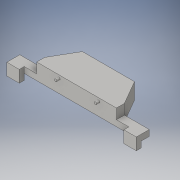
# Autodesk Inventor part: LED_Holder_V1
Saved by Autodesk Inventor 2016 (Build 200138000, 138)
## iProperties
Created: 2016-01-19
Part Number: LED_Holder_V1
Material: Generic
Document SubType Name: Modeling
Designer: Alexis Renderos
Density: 1 g/cm^3
Appearance: Default
Author: Alexis Renderos
Autodesk Inventor part; units mm, degrees
ref_plane "YZ Plane" through (0, 0, 0) normal (1, 0, 0) x (0, 1, 0)
ref_plane "XZ Plane" through (0, 0, 0) normal (0, 1, 0) x (-1, 0, 0)
ref_plane "XY Plane" through (0, 0, 0) normal (0, 0, 1) x (1, 0, 0)
sketch "Sketch1" plane through (0, 0, 0) normal (0, 0, 1) x (1, 0, 0)
  line L0 (0, 12.3444) -> (0, -2.0574) projected
  line L1 (-35.56, 0) -> (35.56, 0) projected
  line L2 (-35.56, 0) -> (35.56, 0) projected
  line L3 (0, -2.0574) -> (0, 12.3444) projected
  line L4 (-12.319, 8.2169) -> (15.113, 8.2169)
  line L5 (-10.2108, 8.2169) -> (13.0048, 8.2169)
  circle A0 centre (-11.2649, 8.2169) radius 1.0541
  circle A1 centre (14.0589, 8.2169) radius 1.0541
  line L6 (-25.4, 10.287) -> (-25.4, 0)
  line L7 (-25.4, 0) -> (25.4, 0)
  line L8 (-25.4, 10.287) -> (25.4, 10.287)
  line L9 (25.4, 10.287) -> (25.4, 0)
  line L10 (25.4, 10.287) -> (14.0589, 10.287)
  line L11 (14.0589, 10.287) -> (14.0589, 7.1628)
  line L12 (14.0589, 9.271) -> (14.0589, 10.287)
  line L13 (14.0589, 8.2169) -> (15.113, 8.2169)
  circle A2 centre (-11.2649, 8.2169) radius 0.8001
  circle A3 centre (14.0589, 8.2169) radius 0.8001
  point P0 (0, 0)
  dimension "d0" = 27.432
  dimension "d1" = 23.2156
  dimension "d2" = 2.1082
  dimension "d3" = 10.287
  dimension "d4" = 50.8
  dimension "d5" = 11.3411
  dimension "d6" = 1.016
  dimension "d7" = 11.3411
  dimension "d8" = 0.254
  dimension "d9" = 0.254
  constraints: 20 end point, 4 centre point, 4 horizontal, 3 perpendicular, 3 point on circle, 3 point on line, 1 equal radius, 1 vertical
  measures "d0" distance of L4.start L4.end
  measures "d1" distance of L5.start L5.end
  measures "d2" diameter of A0
  measures "d3" distance of L6.start L6.end
  measures "d4" distance of L6.end L7.end
  measures "d5" distance of L8.end L10.end
  measures "d6" distance of L12.start L12.end
  measures "d7" distance between parallel lines of L9 L12
  measures "d8" radial gap between concentric circles of A0 A2
  measures "d9" radial gap between concentric circles of A1 A3
extrude "Extrusion1" add sketch "Sketch1" against normal blind 5.08 contours L8 L11 A1 L4 L0 | L0 L1 L6 L8 | L4 A1 L11 L8 L9 L1 L0
extrude "Extrusion2" add sketch "Sketch1" against normal blind 5.08 contours A0 L4 A2 | L4 A2 A0 | A1 L11 A3 L4 | L4 A3 L11 A1 | A1 L4 A3 L11 | A2 L4 | L4 A2 | A3 L11 L4 | L4 L11 A3 | L11 A3 L4 A1 | A3 L4 L11 | L4 A3 L11
extrude "Extrusion3" add sketch "Sketch1" along normal blind 2.032 contours A2 L4 | L4 A2 | A3 L11 L4 | L4 L11 A3 | A3 L4 L11 | L4 A3 L11
sketch "Sketch2" plane through (-25.4, 0, 0) normal (0, -1, 0) x (1, 0, 0)
  line L0 (50.8, 0) -> (50.8, -5.08) projected
  line L1 (0, 0) -> (50.8, 0) projected
  line L2 (0, 0) -> (0, -5.08) projected
  line L3 (38.1, -5.08) -> (12.7, -5.08)
  line L4 (12.7, -17.78) -> (38.1, -17.78)
  arc A0 (38.1, -12.7) -> (38.1, -10.16) centre (38.1, -11.43) ccw
  arc A1 (12.7, -10.16) -> (12.7, -12.7) centre (12.7, -11.43) ccw
  line L5 (38.1, -17.78) -> (38.1, -12.7)
  line L6 (38.1, -10.16) -> (38.1, -5.08)
  line L7 (12.7, -5.08) -> (12.7, -10.16)
  line L8 (12.7, -12.7) -> (12.7, -17.78)
  line L9 (50.8, 0) -> (0, 0)
  line L10 (25.4, 0) -> (25.4, -33.3128)
  line L11 (25.4, -5.08) -> (25.4, -17.78)
  line L12 (50.8, -5.08) -> (0, -5.08) projected
  line L13 (50.8, -5.08) -> (0, -5.08)
  line L14 (50.8, -5.08) -> (42.0012, -20.32)
  line L15 (50.8, -5.08) -> (70.0547, -5.08) construction
  line L16 (0, -5.08) -> (8.7988, -20.32)
  line L17 (0, -5.08) -> (24.702, -5.08) construction
  line L18 (42.0012, -20.32) -> (8.7988, -20.32)
  dimension "d16" = 25.4
  dimension "d17" = 12.7
  dimension "d18" = 2.54
  dimension "d19" = 2.54
  dimension "d20" = 5.08
  dimension "d21" = 5.08
  dimension "d23" = 6.35
  dimension "d24" = 6.35
  dimension "d26" = 120
  dimension "d27" = 60
  dimension "d29" = 12.7
  dimension "d30" = 33.2024
  dimension "d31" = 19.2547
  dimension "d32" = 28.2328
  dimension "d33" = 26.098
  constraints: 30 end point, 6 perpendicular, 5 horizontal, 4 point on circle, 3 midpoint, 2 centre point, 1 collinear, 1 vertical
  measures "d16" distance of L3.start L3.end
  measures "d17" distance of L3.end L4.start
  measures "d18" diameter of A0
  measures "d19" diameter of A1
  measures "d20" distance of L4.end L5.end
  measures "d21" distance of L8.start L4.start
  measures "d23" distance from line of L4 A0.centre
  measures "d24" distance from line of L4 A1.centre
  measures "d26" angle of L14 L15
  measures "d27" angle of L16 L17
  measures "d29" distance between parallel lines of L11 L5
  measures "d30" distance of L14.end L16.end
  measures "d31" distance from line of L15.end L0
  measures "d32" distance from line of L10.end L12
  measures "d33" distance from line of L17.end L0
extrude "Extrusion4" add sketch "Sketch2" against normal blind 10.287 contours L14 L18 L10 L4 L5 A0 L6 L12 | L6 A0 L5 L4 L10 L3 | L10 L4 L8 A1 L7 L3 | L18 L16 L12 L7 A1 L8 L4 L10
extrude "Extrusion5" add sketch "Sketch2" along normal blind 3.81 contours L6 A0 L5 L4 L10 L3 | L10 L4 L8 A1 L7 L3
sketch "Sketch4" plane through (-25.4, 0, 0) normal (0, -1, 0) x (1, 0, 0)
  line L0 (38.1, -5.08) -> (12.7, -5.08)
  line L1 (0, 0) -> (50.8, 0)
  line L2 (0, 0) -> (0, -5.08)
  line L3 (50.8, 0) -> (50.8, -5.08)
  line L4 (-15.875, -5.08) -> (66.675, -5.08)
  line L5 (25.4, 0) -> (25.4, -41.8957)
  line L6 (-15.875, 0) -> (-15.875, -5.08)
  line L7 (0, 0) -> (0, -5.08)
  line L8 (0, 0) -> (-15.875, 0)
  line L9 (0, 0) -> (0, -5.08)
  line L10 (50.8, 0) -> (0, 0)
  line L11 (50.8, 0) -> (50.8, -5.08)
  line L12 (50.8, 0) -> (66.675, 0)
  line L13 (66.675, 0) -> (66.675, -5.08)
  line L14 (-15.875, 0) -> (-15.875, 3.175)
  line L15 (-7.9375, 3.175) -> (-15.875, 3.175)
  line L16 (-7.9375, 3.175) -> (-7.9375, 0)
  line L17 (-15.875, -5.08) -> (-15.875, 3.175)
  line L18 (-15.875, 3.175) -> (-7.9375, 3.175)
  line L19 (-7.9375, 3.175) -> (-7.9375, 0)
  line L20 (50.8, 0) -> (0, 0) projected
  line L21 (-15.875, 0) -> (0, 0)
  line L22 (0, 0) -> (0, -5.08) projected
  line L23 (0, 0) -> (0, -5.08)
  line L24 (0, -5.08) -> (0, 0)
  line L25 (-15.875, -5.08) -> (66.675, -5.08)
  line L26 (25.4, 0) -> (25.4, -5.08)
  line L27 (12.7, -5.08) -> (38.1, -5.08) projected
  line L28 (66.675, 0) -> (66.675, -5.08)
  line L29 (66.675, 0) -> (66.675, 3.175)
  line L30 (58.7375, 3.175) -> (66.675, 3.175)
  line L31 (58.7375, 3.175) -> (58.7375, 0)
  line L32 (50.8, 0) -> (50.8, -5.08)
  line L33 (50.8, 0) -> (50.8, -5.08)
  line L34 (50.8, 0) -> (66.675, 0)
  line L35 (50.8, 0) -> (50.8, -5.08)
  line L36 (50.8, 0) -> (0, 0)
  line L37 (0, 0) -> (50.8, 0)
  line L38 (66.675, -5.08) -> (-15.875, -5.08)
  line L39 (66.675, -5.08) -> (66.675, 3.175)
  line L40 (66.675, 3.175) -> (58.7375, 3.175)
  line L41 (58.7375, 3.175) -> (58.7375, 0)
  line L42 (0, 0) -> (50.8, 0)
  line L43 (66.675, 0) -> (50.8, 0)
  line L44 (50.8, 0) -> (50.8, -5.08)
  line L45 (50.8, 0) -> (50.8, -5.08)
  line L46 (50.8, -5.08) -> (50.8, 0)
  line L47 (66.675, -5.08) -> (-15.875, -5.08)
  line L48 (-15.875, 0) -> (-7.9375, 0)
  dimension "d40" = 82.55
  dimension "d41" = 3.175
  constraints: 92 end point, 9 collinear, 8 symmetric about line, 4 perpendicular, 3 horizontal, 3 vertical, 2 midpoint
  measures "d40" distance of L6.end L4.end
  measures "d41" distance of L6.start L14.end
extrude "Extrusion6" add sketch "Sketch4" against normal blind 3.81 contours L0 L5 L1 L3 L4 | L0 L4 L2 L1 L5 | L3 L12 L13 L4 | L4 L6 L8 L2
extrude "Extrusion7" add sketch "Sketch4" along normal mid plane 7.62 contours L31 L30 L29 L12 | L8 L14 L15 L16
body "Solid1"
